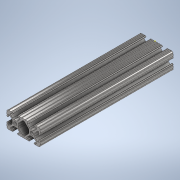
# Autodesk Inventor part: 8 in 2x1 T Slot
Saved by Autodesk Inventor 2020 (Build 240168000, 168)
## iProperties
Created: 2020-01-13
Part Number: 8 in 2x1 T Slot
Material: Steel, Alloy
Document SubType Name: Modeling
Designer: 339294
Density: 7.73 g/cm^3
Appearance: Semi-Polished
Author: 339294
Autodesk Inventor part; units mm, degrees
ref_plane "YZ Plane" through (0, 0, 0) normal (1, 0, 0) x (0, 1, 0)
ref_plane "XZ Plane" through (0, 0, 0) normal (0, 1, 0) x (-1, 0, 0)
ref_plane "XY Plane" through (0, 0, 0) normal (0, 0, 1) x (1, 0, 0)
sketch "Sketch1" plane through (0, 0, 0) normal (0, 0, 1) x (1, 0, 0)
  arc A0 (20.1507, 25.4) -> (21.1667, 25.4) centre (20.6587, 25.4) ccw
  line L0 (20.1507, 25.4) -> (19.1211, 25.4)
  arc A1 (19.1211, 25.4) -> (18.0721, 24.351) centre (19.1211, 24.351) ccw
  line L1 (18.0721, 24.351) -> (18.0721, 24.2392)
  arc A2 (18.0721, 24.2392) -> (19.1211, 23.1902) centre (19.1211, 24.2392) ccw
  line L2 (19.1211, 23.1902) -> (21.25, 23.1902)
  arc A3 (21.9777, 21.4652) -> (21.25, 23.1902) centre (21.25, 22.1742) ccw
  line L3 (21.9777, 21.4652) -> (18.7526, 18.1551)
  arc A4 (16.4785, 17.1958) -> (18.7526, 18.1551) centre (16.4785, 20.3708) ccw
  line L4 (16.4785, 17.1958) -> (13.2169, 17.1958)
  arc A5 (10.9506, 18.1472) -> (13.2169, 17.1958) centre (13.2169, 20.3708) ccw
  line L5 (10.9506, 18.1472) -> (7.6978, 21.4627)
  arc A6 (8.423, 23.1902) -> (7.6978, 21.4627) centre (8.423, 22.1742) ccw
  line L6 (8.423, 23.1902) -> (10.5461, 23.1902)
  arc A7 (10.5461, 23.1902) -> (11.5951, 24.2392) centre (10.5461, 24.2392) ccw
  line L7 (11.5951, 24.2392) -> (11.5951, 24.351)
  arc A8 (11.5951, 24.351) -> (10.5462, 25.4) centre (10.5462, 24.351) ccw
  line L8 (10.5462, 25.4) -> (9.5165, 25.4)
  arc A9 (8.5005, 25.4) -> (9.5165, 25.4) centre (9.0085, 25.4) ccw
  line L9 (8.5005, 25.4) -> (5.2832, 25.4)
  arc A10 (4.2672, 25.4) -> (5.2832, 25.4) centre (4.7752, 25.4) ccw
  line L10 (4.2672, 25.4) -> (0, 25.4)
  arc A11 (-1.016, 25.4) -> (0, 25.4) centre (-0.508, 25.4) ccw
  line L11 (-1.016, 25.4) -> (-4.2333, 25.4)
  arc A12 (-5.2493, 25.4) -> (-4.2333, 25.4) centre (-4.7413, 25.4) ccw
  line L12 (-5.2493, 25.4) -> (-6.2789, 25.4)
  arc A13 (-6.2789, 25.4) -> (-7.3279, 24.351) centre (-6.2789, 24.351) ccw
  line L13 (-7.3279, 24.351) -> (-7.3279, 24.2392)
  arc A14 (-7.3279, 24.2392) -> (-6.2789, 23.1902) centre (-6.2789, 24.2392) ccw
  line L14 (-6.2789, 23.1902) -> (-4.15, 23.1902)
  arc A15 (-3.399, 21.3661) -> (-4.15, 23.1902) centre (-4.15, 22.1235) ccw
  line L15 (-3.399, 21.3661) -> (-6.6764, 18.1163)
  arc A16 (-8.9119, 17.1958) -> (-6.6764, 18.1163) centre (-8.9119, 20.3708) ccw
  line L16 (-8.9119, 17.1958) -> (-12.2209, 17.1958)
  arc A17 (-14.4564, 18.1163) -> (-12.2209, 17.1958) centre (-12.2209, 20.3708) ccw
  line L17 (-14.4564, 18.1163) -> (-17.7338, 21.3661)
  arc A18 (-16.9828, 23.1902) -> (-17.7338, 21.3661) centre (-16.9828, 22.1235) ccw
  line L18 (-16.9828, 23.1902) -> (-14.8539, 23.1902)
  arc A19 (-14.8539, 23.1902) -> (-13.8049, 24.2392) centre (-14.8539, 24.2392) ccw
  line L19 (-13.8049, 24.2392) -> (-13.8049, 24.351)
  arc A20 (-13.8049, 24.351) -> (-14.8538, 25.4) centre (-14.8538, 24.351) ccw
  line L20 (-14.8538, 25.4) -> (-15.8835, 25.4)
  arc A21 (-16.8995, 25.4) -> (-15.8835, 25.4) centre (-16.3915, 25.4) ccw
  line L21 (-16.8995, 25.4) -> (-20.1168, 25.4)
  arc A22 (-21.1328, 25.3998) -> (-20.1168, 25.4) centre (-20.6248, 25.4) ccw
  arc A23 (-21.1328, 25.3998) -> (-23.2662, 23.2664) centre (-21.1582, 23.2918) ccw
  arc A24 (-23.2664, 22.2504) -> (-23.2662, 23.2664) centre (-23.2664, 22.7584) ccw
  line L22 (-23.2664, 22.2504) -> (-23.2664, 19.0331)
  arc A25 (-23.2664, 18.0171) -> (-23.2664, 19.0331) centre (-23.2664, 18.5251) ccw
  line L23 (-23.2664, 18.0171) -> (-23.2664, 16.9375)
  arc A26 (-23.2664, 16.9375) -> (-22.2674, 15.9385) centre (-22.2674, 16.9375) ccw
  line L24 (-22.2674, 15.9385) -> (-22.1056, 15.9385)
  arc A27 (-22.1056, 15.9385) -> (-21.0566, 16.9875) centre (-22.1056, 16.9875) ccw
  line L25 (-21.0566, 16.9875) -> (-21.0566, 19.0347)
  arc A28 (-19.3004, 19.7665) -> (-21.0566, 19.0347) centre (-20.026, 19.0347) ccw
  line L26 (-19.3004, 19.7665) -> (-16.0143, 16.5082)
  arc A29 (-15.0749, 14.2536) -> (-16.0143, 16.5082) centre (-18.2499, 14.2536) ccw
  line L27 (-15.0749, 14.2536) -> (-15.0749, 11.0048)
  arc A30 (-16.0069, 8.7577) -> (-15.0749, 11.0048) centre (-18.2499, 11.0048) ccw
  line L28 (-16.0069, 8.7577) -> (-19.298, 5.4726)
  arc A31 (-21.0566, 6.202) -> (-19.298, 5.4726) centre (-20.026, 6.202) ccw
  line L29 (-21.0566, 6.202) -> (-21.0566, 8.4125)
  arc A32 (-21.0566, 8.4125) -> (-22.1056, 9.4615) centre (-22.1056, 8.4125) ccw
  line L30 (-22.1056, 9.4615) -> (-22.2174, 9.4615)
  arc A33 (-22.2174, 9.4615) -> (-23.2664, 8.4125) centre (-22.2174, 8.4125) ccw
  line L31 (-23.2664, 8.4125) -> (-23.2664, 7.3829)
  arc A34 (-23.2664, 6.3669) -> (-23.2664, 7.3829) centre (-23.2664, 6.8749) ccw
  line L32 (-23.2664, 6.3669) -> (-23.2664, 3.1496)
  arc A35 (-23.2662, 2.1336) -> (-23.2664, 3.1496) centre (-23.2664, 2.6416) ccw
  arc A36 (-23.2662, 2.1336) -> (-21.1328, 0.0002) centre (-21.1582, 2.1082) ccw
  arc A37 (-20.1168, 0) -> (-21.1328, 0.0002) centre (-20.6248, 0) ccw
  line L33 (-20.1168, 0) -> (-16.8995, 0)
  arc A38 (-15.8835, 0) -> (-16.8995, 0) centre (-16.3915, 0) ccw
  line L34 (-15.8835, 0) -> (-14.8539, 0)
  arc A39 (-14.8539, 0) -> (-13.8048, 1.049) centre (-14.8539, 1.049) ccw
  line L35 (-13.8048, 1.049) -> (-13.8048, 1.1608)
  arc A40 (-13.8048, 1.1608) -> (-14.8539, 2.2098) centre (-14.8539, 1.1608) ccw
  line L36 (-14.8539, 2.2098) -> (-16.9828, 2.2098)
  arc A41 (-17.7005, 3.9449) -> (-16.9828, 2.2098) centre (-16.9828, 3.2258) ccw
  line L37 (-17.7005, 3.9449) -> (-14.363, 7.2763)
  arc A42 (-12.12, 8.2042) -> (-14.363, 7.2763) centre (-12.12, 5.0292) ccw
  line L38 (-12.12, 8.2042) -> (-9.0128, 8.2042)
  arc A43 (-6.7698, 7.2763) -> (-9.0128, 8.2042) centre (-9.0128, 5.0292) ccw
  line L39 (-6.7698, 7.2763) -> (-3.4323, 3.9449)
  arc A44 (-4.15, 2.2098) -> (-3.4323, 3.9449) centre (-4.15, 3.2258) ccw
  line L40 (-4.15, 2.2098) -> (-6.2789, 2.2098)
  arc A45 (-6.2789, 2.2098) -> (-7.3279, 1.1608) centre (-6.2789, 1.1608) ccw
  line L41 (-7.3279, 1.1608) -> (-7.3279, 1.049)
  arc A46 (-7.3279, 1.049) -> (-6.2789, 0) centre (-6.2789, 1.049) ccw
  line L42 (-6.2789, 0) -> (-5.2493, 0)
  arc A47 (-4.2333, 0) -> (-5.2493, 0) centre (-4.7413, 0) ccw
  line L43 (-4.2333, 0) -> (-1.016, 0)
  arc A48 (0, 0) -> (-1.016, 0) centre (-0.508, 0) ccw
  line L44 (0, 0) -> (4.2672, 0)
  arc A49 (5.2832, 0) -> (4.2672, 0) centre (4.7752, 0) ccw
  line L45 (5.2832, 0) -> (8.5005, 0)
  arc A50 (9.5165, 0) -> (8.5005, 0) centre (9.0085, 0) ccw
  line L46 (9.5165, 0) -> (10.5461, 0)
  arc A51 (10.5461, 0) -> (11.5952, 1.049) centre (10.5461, 1.049) ccw
  line L47 (11.5952, 1.049) -> (11.5952, 1.1608)
  arc A52 (11.5952, 1.1608) -> (10.5461, 2.2098) centre (10.5461, 1.1608) ccw
  line L48 (10.5461, 2.2098) -> (8.423, 2.2098)
  arc A53 (7.6143, 4.1647) -> (8.423, 2.2098) centre (8.423, 3.3545) ccw
  line L49 (7.6143, 4.1647) -> (10.7315, 7.2763)
  arc A54 (12.9746, 8.2042) -> (10.7315, 7.2763) centre (12.9746, 5.0292) ccw
  line L50 (12.9746, 8.2042) -> (16.2362, 8.2042)
  arc A55 (18.3215, 7.4234) -> (16.2362, 8.2042) centre (16.2362, 5.0292) ccw
  line L51 (18.3215, 7.4234) -> (22.0019, 4.2178)
  arc A56 (21.25, 2.2098) -> (22.0019, 4.2178) centre (21.25, 3.3545) ccw
  line L52 (21.25, 2.2098) -> (19.1211, 2.2098)
  arc A57 (19.1211, 2.2098) -> (18.0721, 1.1608) centre (19.1211, 1.1608) ccw
  line L53 (18.0721, 1.1608) -> (18.0721, 1.049)
  arc A58 (18.0721, 1.049) -> (19.1211, 0) centre (19.1211, 1.049) ccw
  line L54 (19.1211, 0) -> (20.1507, 0)
  arc A59 (21.1667, 0) -> (20.1507, 0) centre (20.6587, 0) ccw
  line L55 (21.1667, 0) -> (24.384, 0)
  arc A60 (25.4, 0.0002) -> (24.384, 0) centre (24.892, 0) ccw
  arc A61 (25.4, 0.0002) -> (27.5335, 2.1336) centre (25.4254, 2.1082) ccw
  arc A62 (27.5336, 3.1496) -> (27.5335, 2.1336) centre (27.5336, 2.6416) ccw
  line L56 (27.5336, 3.1496) -> (27.5336, 6.3669)
  arc A63 (27.5336, 7.3829) -> (27.5336, 6.3669) centre (27.5336, 6.8749) ccw
  line L57 (27.5336, 7.3829) -> (27.5336, 8.4625)
  arc A64 (27.5336, 8.4625) -> (26.5346, 9.4615) centre (26.5346, 8.4625) ccw
  line L58 (26.5346, 9.4615) -> (26.3228, 9.4615)
  arc A65 (26.3228, 9.4615) -> (25.3238, 8.4625) centre (26.3228, 8.4625) ccw
  line L59 (25.3238, 8.4625) -> (25.3238, 6.5441)
  arc A66 (23.7176, 5.8131) -> (25.3238, 6.5441) centre (24.3543, 6.5441) ccw
  line L60 (23.7176, 5.8131) -> (20.4318, 8.675)
  arc A67 (19.3421, 11.0692) -> (20.4318, 8.675) centre (22.5171, 11.0692) ccw
  line L61 (19.3421, 11.0692) -> (19.3421, 14.3308)
  arc A68 (20.243, 16.5465) -> (19.3421, 14.3308) centre (22.5171, 14.3308) ccw
  line L62 (20.243, 16.5465) -> (23.66, 20.0534)
  arc A69 (25.3238, 19.3769) -> (23.66, 20.0534) centre (24.3543, 19.3769) ccw
  line L63 (25.3238, 19.3769) -> (25.3238, 16.9375)
  arc A70 (25.3238, 16.9375) -> (26.3228, 15.9385) centre (26.3228, 16.9375) ccw
  line L64 (26.3228, 15.9385) -> (26.5346, 15.9385)
  arc A71 (26.5346, 15.9385) -> (27.5336, 16.9375) centre (26.5346, 16.9375) ccw
  line L65 (27.5336, 16.9375) -> (27.5336, 18.0171)
  arc A72 (27.5336, 19.0332) -> (27.5336, 18.0171) centre (27.5336, 18.5251) ccw
  line L66 (27.5336, 19.0332) -> (27.5336, 22.2504)
  arc A73 (27.5335, 23.2664) -> (27.5336, 22.2504) centre (27.5336, 22.7584) ccw
  arc A74 (27.5335, 23.2664) -> (25.4, 25.3998) centre (25.4254, 23.2918) ccw
  arc A75 (24.384, 25.4) -> (25.4, 25.3998) centre (24.892, 25.4) ccw
  line L67 (24.384, 25.4) -> (21.1667, 25.4)
  line L68 (1.7004, 2.667) -> (2.5668, 2.667)
  arc A76 (0.5879, 3.1272) -> (1.7004, 2.667) centre (1.7004, 4.2418) ccw
  line L69 (-5.1259, 8.8306) -> (0.5879, 3.1272)
  arc A77 (-6.0579, 11.0777) -> (-5.1259, 8.8306) centre (-2.8829, 11.0777) ccw
  line L70 (-6.0579, 14.3223) -> (-6.0579, 11.0777)
  arc A78 (-5.1184, 16.5768) -> (-6.0579, 14.3223) centre (-2.8829, 14.3223) ccw
  line L71 (0.6296, 22.2765) -> (-5.1184, 16.5768)
  arc A79 (1.7384, 22.733) -> (0.6296, 22.2765) centre (1.7384, 21.1582) ccw
  line L72 (2.6851, 22.733) -> (1.7384, 22.733)
  arc A80 (3.8092, 22.2611) -> (2.6851, 22.733) centre (2.6851, 21.1582) ccw
  line L73 (9.4165, 16.5459) -> (3.8092, 22.2611)
  arc A81 (10.3251, 14.3223) -> (9.4165, 16.5459) centre (7.1501, 14.3223) ccw
  line L74 (10.3251, 11.0777) -> (10.3251, 14.3223)
  arc A82 (9.3931, 8.8306) -> (10.3251, 11.0777) centre (7.1501, 11.0777) ccw
  line L75 (3.6794, 3.1272) -> (9.3931, 8.8306)
  arc A83 (2.5668, 2.667) -> (3.6794, 3.1272) centre (2.5668, 4.2418) ccw
  circle A84 centre (14.8336, 12.7) radius 2.6035
  circle A85 centre (-10.5664, 12.7) radius 2.6035
  point P0 (2.1336, 12.7)
  constraints: 168 point on circle, 152 end point, 86 centre point
extrude "Extrusion1" add sketch "Sketch1" along normal blind 203.2
sketch "Sketch2" plane through (0, 25.4, 0) normal (0, 1, 0) x (1, 0, 0)
  point P0 (0, 0)
body "Solid1"
